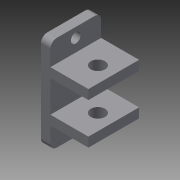
# Autodesk Inventor part: support_clip_base(2)
Saved by Autodesk Inventor 2015 (Build 190159000, 159)
## iProperties
Created: 2017-10-02
Part Number: support_clip_base(2)
Material: Generic
Document SubType Name: Modeling
Designer: Anshul
Density: 1 g/cm^3
Appearance: Default
Author: Anshul
Autodesk Inventor part; units mm, degrees
ref_plane "YZ Plane" through (0, 0, 0) normal (1, 0, 0) x (0, 1, 0)
ref_plane "XZ Plane" through (0, 0, 0) normal (0, 1, 0) x (-1, 0, 0)
ref_plane "XY Plane" through (0, 0, 0) normal (0, 0, 1) x (1, 0, 0)
sketch "Sketch1" plane through (0, 0, 0) normal (0, 1, 0) x (-1, 0, 0)
  line L0 (0, 0) -> (0, -280)
  line L1 (0, -280) -> (17, -280)
  line L2 (17, -280) -> (17, 0)
  line L3 (17, 0) -> (0, 0)
  line L4 (0, 0) -> (-10, 0)
  line L5 (-10, 0) -> (-10, -40)
  line L6 (-10, -40) -> (0, -40)
  line L7 (0, 0) -> (0, -125)
  line L8 (0, 0) -> (-70, 0)
  line L9 (0, -125) -> (0, -145)
  line L10 (0, -145) -> (0, -165)
  line L11 (-70, 0) -> (0, -145)
  circle A0 centre (-70, 0) radius 12.5
  line L12 (-81.2569, -5.4344) -> (0, -173.7522)
  line L13 (-70, 0) -> (-58.7431, 5.4344)
  line L14 (-58.7431, 5.4344) -> (0, -116.2478)
  line L15 (-70, 0) -> (-70, -3.2)
  line L16 (-81.2569, -5.4344) -> (-83.8804, 0)
  line L17 (-64.5656, -11.2569) -> (-64.5656, 0)
  line L18 (-64.5656, 0) -> (-76.5656, 0)
  line L19 (-64.5656, 0) -> (-52.5656, 0)
  line L20 (-64.5656, -11.2569) -> (-64.5656, -19.2569)
  line L21 (-64.5656, -19.2569) -> (-76.5656, -19.2569)
  line L22 (-76.5656, -19.2569) -> (-76.5656, 0)
  line L23 (-64.5656, -19.2569) -> (-52.5656, -19.2569)
  line L24 (-52.5656, -19.2569) -> (-52.5656, 0)
  line L25 (-70, -3.2) -> (-76.5656, -3.2)
  line L26 (-70, -3.2) -> (-52.5656, -3.2)
  line L27 (-52.5656, -3.2) -> (-52.5656, -6.2)
  line L28 (-52.5656, -6.2) -> (-76.5656, -6.2)
  line L29 (-64.5656, -6.2) -> (-64.5656, -12.2)
  circle A1 centre (-64.5656, -12.2) radius 2.4
  line L30 (0, -145) -> (0, -157)
  line L31 (0, -145) -> (0, -133)
  line L32 (0, -145) -> (-3, -145)
  line L33 (-3, -145) -> (-10, -145)
  circle A2 centre (-10, -145) radius 2.25
  line L34 (0, -145) -> (0, -137)
  line L35 (0, -137) -> (-15, -137)
  line L36 (-15, -137) -> (-15, -145)
  line L37 (0, -145) -> (0, -153)
  line L38 (0, -153) -> (-15, -153)
  line L39 (-15, -153) -> (-15, -145)
  line L40 (-3, -145) -> (-3, -137)
  line L41 (-3, -145) -> (-3, -153)
  dimension "d0" = 280
  dimension "d1" = 17
  dimension "d2" = 280
  dimension "d3" = 10
  dimension "d4" = 40
  dimension "d5" = 125
  dimension "d6" = 70
  dimension "d7" = 20
  dimension "d8" = 20
  dimension "d10" = 25
  dimension "d11" = 3.2
  dimension "d12" = 12
  dimension "d13" = 12
  dimension "d14" = 8
  dimension "d16" = 3
  dimension "d17" = 6
  dimension "d18" = 4.8
  dimension "d19" = 12
  dimension "d20" = 12
  dimension "d21" = 3
  dimension "d22" = 7
  dimension "d23" = 4.5
  dimension "d24" = 5
  dimension "d25" = 8
  dimension "d26" = 8
  constraints: 84 end point, 28 point on line, 18 perpendicular, 3 centre point, 3 coincident, 3 point on circle, 2 parallel, 2 vertical, 1 collinear, 1 midpoint
  measures "d0" distance of L0.start L0.end
  measures "d1" distance of L0.end L1.end
  measures "d2" distance of L1.end L2.end
  measures "d3" distance of L0.start L4.end
  measures "d4" distance of L4.end L5.end
  measures "d5" distance of L0.start L7.end
  measures "d6" distance of L0.start L8.end
  measures "d7" distance of L7.end L9.end
  measures "d8" distance of L9.end L10.end
  measures "d10" diameter of A0
  measures "d11" distance of L13.start L15.end
  measures "d12" distance of L17.end L18.end
  measures "d13" distance of L17.end L19.end
  measures "d14" distance of L17.start L20.end
  measures "d16" distance of L26.end L27.end
  measures "d17" distance of L29.start L29.end
  measures "d18" diameter of A1
  measures "d19" distance of L9.end L30.end
  measures "d20" distance of L9.end L31.end
  measures "d21" distance of L9.end L32.end
  measures "d22" distance of L32.end L33.end
  measures "d23" diameter of A2
  measures "d24" distance of A2.centre L36.end
  measures "d25" distance of L9.end L34.end
  measures "d26" distance of L9.end L37.end
extrude "Extrusion1" add sketch "Sketch1" along normal mid plane 16 contours L0 L11 L40 L35 | L38 L39 L36 L12 | L12 L36 L35 L11 L40 L41 L38 | L32 L40 L11 | L0 L38 L41 L32 | L40 L11 L35
extrude "Extrusion2" cut sketch "Sketch1" along normal mid plane 10 contours L38 L39 L36 L12 | L12 L36 L35 L11 L40 L41 L38 | L40 L11 L35
extrude "Extrusion3" add sketch "Sketch1" along normal mid plane 30 contours L0 L11 L40 L35 | L32 L40 L11 | L0 L38 L41 L32
sketch "Sketch2" plane through (0, -15, -153) normal (-1, 0, 0) x (0, 0, 1)
  line L0 (0, 23) -> (0, 30)
  line L1 (0, 0) -> (0, 30) projected
  line L2 (0, 30) -> (8, 30)
  line L3 (16, 30) -> (0, 30) projected
  line L4 (8, 30) -> (8, 27)
  circle A0 centre (8, 27) radius 1.55
  line L5 (0, 0) -> (8, 0)
  line L6 (8, 0) -> (8, 3)
  circle A1 centre (8, 3) radius 1.55
  point P0 (153, 15)
  dimension "d33" = 8
  dimension "d34" = 3
  dimension "d35" = 3.1
  dimension "d36" = 8
  dimension "d37" = 3
  dimension "d38" = 3.1
  constraints: 10 end point, 2 centre point, 2 coincident, 2 perpendicular, 1 collinear, 1 horizontal, 1 midpoint
  measures "d33" distance of L0.end L2.end
  measures "d34" distance of L2.end L4.end
  measures "d35" diameter of A0
  measures "d36" distance of L1.start L5.end
  measures "d37" distance of L5.end L6.end
  measures "d38" diameter of A1
extrude "Extrusion4" cut sketch "Sketch2" against normal blind 30
fillet "Fillet1" radius 2 4 edges at (1.5, 15, -153) (1.5, -15, -153) (1.5, -15, -137) (1.5, 15, -137)
body "Solid1"
